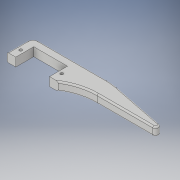
# Autodesk Inventor part: tibia_v3
Saved by Autodesk Inventor 2019 (Build 230136000, 136)
## iProperties
Created: 2018-12-28
Part Number: tibia_v3
Material: Generic
Document SubType Name: Modeling
Designer: Daniel
Density: 1 g/cm^3
Appearance: Default
Author: Daniel
Autodesk Inventor part; units mm, degrees
ref_plane "YZ Plane" through (0, 0, 0) normal (1, 0, 0) x (0, 1, 0)
ref_plane "XZ Plane" through (0, 0, 0) normal (0, 1, 0) x (-1, 0, 0)
ref_plane "XY Plane" through (0, 0, 0) normal (0, 0, 1) x (1, 0, 0)
sketch "Sketch1" plane through (0, 0, 0) normal (0, 1, 0) x (-1, 0, 0)
  line L0 (0, -12.6) -> (0, 12.6) projected
  line L1 (35.5, -9) -> (0, -9)
  line L2 (0, -9) -> (0, 9)
  line L3 (0, 9) -> (35.5, 9)
  line L4 (35.5, 9) -> (35.5, -9)
  line L5 (0, 0) -> (0, -9)
  line L6 (0, 0) -> (0, -9)
  line L7 (55.6, 0) -> (-85.1, 0) projected
  line L8 (0, -9) -> (-65, -9)
  line L9 (-65, -9) -> (-65, 3)
  line L10 (-65, 3) -> (0, 3)
  line L11 (0, 3) -> (0, -9)
  point P0 (0, 0)
  dimension "d53" = 18
  dimension "d54" = 35.5
  dimension "d56" = 6
  dimension "d57" = 65
  constraints: 20 end point, 4 collinear, 4 parallel, 2 horizontal, 2 perpendicular, 1 other
  measures "d53" distance between parallel lines of L3 L1
  measures "d54" distance between parallel lines of L2 L4
  measures "d56" distance between parallel lines of L3 L10
  measures "d57" distance between parallel lines of L9 L0
extrude "Extrusion3" add sketch "Sketch1" along normal blind 6
sketch "Sketch4" plane through (0, 6, 0) normal (0, 1, 0) x (1, 0, 0)
  line L0 (-35.5, 9) -> (-35.5, -9) projected
  line L1 (-35.5, -9) -> (0, -9) projected
  line L2 (0, -9) -> (0, -3) projected
  line L3 (0, -3) -> (65, -3) projected
  line L4 (65, -3) -> (65, 9) projected
  line L5 (65, 9) -> (-35.5, 9) projected
  line L6 (0, 12.6) -> (0, -12.6) projected
  line L7 (-55.6, 0) -> (85.1, 0) projected
  line L8 (-29.5, 3.5) -> (-6, 3.5)
  line L9 (-6, 3.5) -> (-6, -9)
  line L10 (-6, -9) -> (-29.5, -9)
  line L11 (-29.5, -9) -> (-29.5, 3.5)
  line L12 (-35.5, -9) -> (0, -9) projected
  line L13 (65, 9) -> (-35.5, 9) projected
  line L14 (20, 9) -> (65, 0)
  point P0 (0, 0)
  point P1 (0, 9)
  dimension "d58" = 23.5
  dimension "d59" = 12.5
  dimension "d60" = 6
  dimension "d64" = 20
  constraints: 10 end point, 5 point on line, 2 parallel, 1 collinear, 1 horizontal, 1 perpendicular
  measures "d58" distance between parallel lines of L9 L11
  measures "d59" distance between parallel lines of L10 L8
  measures "d60" distance between parallel lines of L0 L11
  measures "d64" distance from line of L6 L14.start
extrude "Extrusion5" cut sketch "Sketch4" against normal up to next contours L11 L8 L9 L7 | L7 L9 L1 L11 | L5 L4 L14
fillet "Fillet10" radius 40 2 edges at (0, 3, 3) (20, 3, -9)
fillet "Fillet11" radius 2 2 edges at (65, 3, 0) (65, 3, 3)
sketch "Sketch5" plane through (0, 6, 0) normal (0, 1, 0) x (1, 0, 0)
  arc A0 (59.802, -3) -> (60.1942, 0.9612) centre (59.802, -1) ccw projected
  line L0 (60.1942, 0.9612) -> (23.8839, 8.2232) projected
  arc A1 (23.8839, 8.2232) -> (16.0392, 9) centre (16.0392, -31) ccw projected
  line L1 (16.0392, 9) -> (-35.5, 9) projected
  line L2 (-35.5, 9) -> (-35.5, -9) projected
  line L3 (-35.5, -9) -> (-29.5, -9) projected
  line L4 (-29.5, -9) -> (-29.5, 3.5) projected
  line L5 (-29.5, 3.5) -> (-6, 3.5) projected
  line L6 (-6, 3.5) -> (-6, -9) projected
  line L7 (-6, -9) -> (0, -9) projected
  arc A2 (21.0713, -3) -> (0, -9) centre (21.0713, -43) ccw projected
  line L8 (21.0713, -3) -> (59.802, -3) projected
  line L9 (0, 19.6325) -> (0, -53.4387) projected
  line L10 (-55.6, 0) -> (85.1, 0) projected
  point P0 (0, 0)
  point P1 (-32, -3)
  point P2 (-3.5, -3)
  dimension "d69" = 6
  dimension "d70" = 6
  dimension "d71" = 2.5
  dimension "d72" = 2.5
  measures "d69" distance from line of L3 point (-32, -3)
  measures "d70" distance from line of L7 point (-3.5, -3)
  measures "d71" distance from line of L6 point (-3.5, -3)
  measures "d72" distance from line of L4 point (-32, -3)
hole "Hole3" at (-32, 6, 3) at (-3.5, 6, 3) direction (0, -1, 0) diameter 2 depth 2.5
fillet "Fillet12" radius 4 1 edges at (-35.5, 3, -9)
fillet "Fillet13" radius 1 14 edges at (19.9807, 0, -8.8053) (40.4371, 0, 3) (61.7931, 0, 1.1972) (42.0395, 0, -4.5921) (-7.7304, 0, -9) (-34.3284, 0, -7.8284) (-35.5, 0, 2) (-34.3284, 6, -7.8284) (-35.5, 6, 2) (19.9807, 6, -8.8053) (42.0395, 6, -4.5921) (61.7931, 6, 1.1972) (40.4371, 6, 3) (-7.7304, 6, -9)
body "Solid3"
